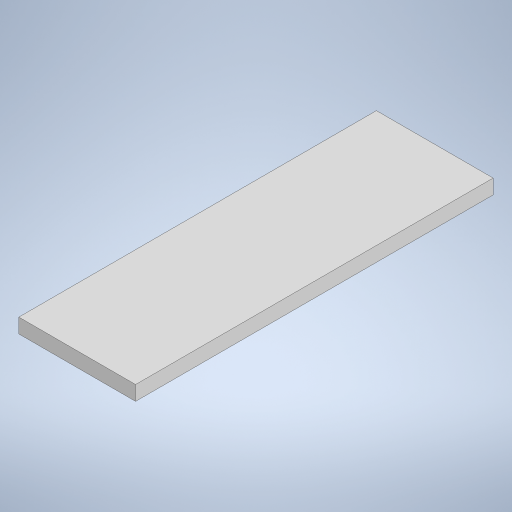
# Autodesk Inventor part: front_2
Saved by Autodesk Inventor 2023 (Build 270158000, 158)
## iProperties
Created: 2024-04-26
Part Number: front_2
Material: 常规
Document SubType Name: Modeling
Designer: Nitrene.P.L
Density: 1 g/cm^3
Appearance: 默认
Author: Nitrene.P.L
Autodesk Inventor part; units mm, degrees
ref_plane "YZ Plane" through (0, 0, 0) normal (1, 0, 0) x (0, 1, 0)
ref_plane "XZ Plane" through (0, 0, 0) normal (0, 1, 0) x (-1, 0, 0)
ref_plane "XY Plane" through (0, 0, 0) normal (0, 0, 1) x (1, 0, 0)
sketch "草图1" plane through (0, 0, 0) normal (0, 1, 0) x (-1, 0, 0)
  line L0 (40, 245) -> (-40, 245)
  line L1 (-40, 245) -> (-40, -245)
  line L2 (-40, -245) -> (40, -245)
  line L3 (40, -245) -> (40, 245)
  line L4 (0, 5.532) -> (0, -5.7915)
  line L5 (3, 0) -> (-2, 0)
  line L6 (40, 0) -> (-40, 0)
  point P0 (0, 0)
  point P1 (0, 0)
  point P2 (0, 0)
  point P3 (-2, 0)
  dimension "d0" = 80
  dimension "d1" = 490
  constraints: 14 end point, 2 horizontal, 2 midpoint, 2 parallel, 2 vertical, 1 perpendicular, 2 other
  measures "d0" distance of L2.end L1.end
  measures "d1" distance of L1.end L0.end
extrude "拉伸1" add sketch "草图1" along normal blind 10 contours L3 L2 L1 L6 L5
